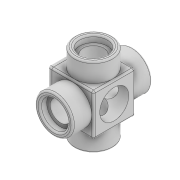
# Autodesk Inventor part: Cross
Saved by Autodesk Inventor 2020 (Build 240168000, 168)
## iProperties
Created: 2021-04-25
Part Number: Cross
Material: Generic
Document SubType Name: Modeling
Designer: deox
Density: 1 g/cm^3
Appearance: Default
Author: deox
Autodesk Inventor part; units mm, degrees
ref_plane "YZ Plane" through (0, 0, 0) normal (1, 0, 0) x (0, 1, 0)
ref_plane "XZ Plane" through (0, 0, 0) normal (0, 1, 0) x (-1, 0, 0)
ref_plane "XY Plane" through (0, 0, 0) normal (0, 0, 1) x (1, 0, 0)
sketch "Sketch1" plane through (0, 0, 0) normal (0, 0, 1) x (1, 0, 0)
  line L0 (-3, -3) -> (3, -3)
  line L1 (3, -3) -> (3, 3)
  line L2 (3, 3) -> (-3, 3)
  line L3 (-3, 3) -> (-3, -3)
  line L4 (-3, -3) -> (3, 3) construction
  line L5 (3, -3) -> (-3, 3) construction
  point P0 (0, 0)
  dimension "d0" = 6
  dimension "d1" = 6
  constraints: 12 end point, 2 midpoint, 2 parallel, 1 horizontal, 1 perpendicular
  measures "d0" distance of L2.end L1.end
  measures "d1" distance of L1.end L0.end
extrude "Extrusion1" add sketch "Sketch1" along normal mid plane 6
sketch "Sketch2" plane through (-3, 3, 3) normal (0, 1, 0) x (1, 0, 0)
  circle A0 centre (3, 3) radius 2.75
  dimension "d4" = 5.5
  constraints: 1 centre point, 1 coincident
  measures "d4" diameter of A0
extrude "Extrusion2" add sketch "Sketch2" along normal blind 2.75
sketch "Sketch3" plane through (-3, -3, 3) normal (0, -1, 0) x (1, 0, 0)
  circle A0 centre (3, -3) radius 2.75
  dimension "d7" = 5.5
  constraints: 1 centre point, 1 coincident
  measures "d7" diameter of A0
extrude "Extrusion3" add sketch "Sketch3" along normal blind 2.75
sketch "Sketch4" plane through (0, 0, -3) normal (0, 0, -1) x (-1, 0, 0)
  circle A0 centre (0, 0) radius 2.75
  dimension "d10" = 5.5
  constraints: 1 centre point, 1 coincident
  measures "d10" diameter of A0
extrude "Extrusion4" add sketch "Sketch4" along normal blind 2.75
sketch "Sketch5" plane through (0, 0, 3) normal (0, 0, 1) x (1, 0, 0)
  circle A0 centre (0, 0) radius 2.75
  dimension "d13" = 5.5
  constraints: 1 centre point, 1 coincident
  measures "d13" diameter of A0
extrude "Extrusion5" add sketch "Sketch5" along normal blind 2.75
sketch "Sketch8" plane through (0, -5.75, 0) normal (0, -1, 0) x (1, 0, 0)
  circle A0 centre (0, 0) radius 1.5
  dimension "d23" = 3
  constraints: 1 centre point, 1 coincident
  measures "d23" diameter of A0
extrude "Extrusion7" cut sketch "Sketch8" against normal through all
sketch "Sketch9" plane through (0, 0, -5.75) normal (0, 0, -1) x (-1, 0, 0)
  circle A0 centre (0, 0) radius 1.5
  dimension "d26" = 3
  constraints: 1 centre point, 1 coincident
  measures "d26" diameter of A0
extrude "Extrusion8" cut sketch "Sketch9" against normal through all
sketch "Sketch10" plane through (0, 5.75, 0) normal (0, 1, 0) x (1, 0, 0)
  circle A0 centre (0, 0) radius 2
  dimension "d30" = 4
  constraints: 1 centre point, 1 coincident
  measures "d30" diameter of A0
extrude "Extrusion9" cut sketch "Sketch10" against normal blind 1
sketch "Sketch11" plane through (0, 0, -5.75) normal (0, 0, -1) x (-1, 0, 0)
  circle A0 centre (0, 0) radius 2
  dimension "d33" = 4
  constraints: 1 centre point, 1 coincident
  measures "d33" diameter of A0
extrude "Extrusion10" cut sketch "Sketch11" against normal blind 1
mirror "Mirror1" about plane through (0, 0, 0) normal (0, 1, 0) of "Extrusion9"
mirror "Mirror2" about plane through (0, 0, 0) normal (0, 0, 1) of "Extrusion10"
sketch "Sketch12" plane through (-3, -3, 3) normal (-1, 0, 0) x (0, 0, 1)
  line L0 (-6, 0) -> (0, 0) projected
  line L1 (0, 6) -> (0, 0) projected
  line L2 (0, 6) -> (-6, 6) projected
  line L3 (-6, 0) -> (-6, 6) projected
  point P0 (-3, 3)
extrude "Extrusion11" add sketch "Sketch12" along normal blind 1
sketch "Sketch13" plane through (3, -3, 3) normal (1, 0, 0) x (0, 0, -1)
  line L0 (3, 3) -> (4.5, 4.5) projected
  circle A0 centre (3, 3) radius 2.1
  dimension "d38" = 4.2
  constraints: 1 centre point, 1 coincident
  measures "d38" diameter of A0
extrude "Extrusion12" cut sketch "Sketch13" against normal blind 5.5
fillet "Fillet4" radius 0.25 8 edges at (-2.75, 0, 5.75) (2, 0, 5.75) (-2.75, 5.75, 0) (-2, 5.75, 0) (2.75, 0, -5.75) (2, 0, -5.75) (-2.75, -5.75, 0) (-2, -5.75, 0)
fillet "Fillet5" radius 0.25 8 edges at (3, 0, -3) (3, 3, 0) (3, 0, 3) (3, -3, 0) (-0.5, 3, -3) (-0.5, 3, 3) (-0.5, -3, -3) (-0.5, -3, 3)
fillet "Fillet6" radius 1 8 edges at (-4, -2.9268, -2.9268) (-4, -3, 0) (-4, -2.9268, 2.9268) (-4, 0, 3) (-4, 2.9268, 2.9268) (-4, 3, 0) (-4, 2.9268, -2.9268) (-4, 0, -3)
ref_plane "Work Plane1" through (0, 0, 0) normal (0, 1, 0) x (-1, 0, 0)
body "Solid1"
